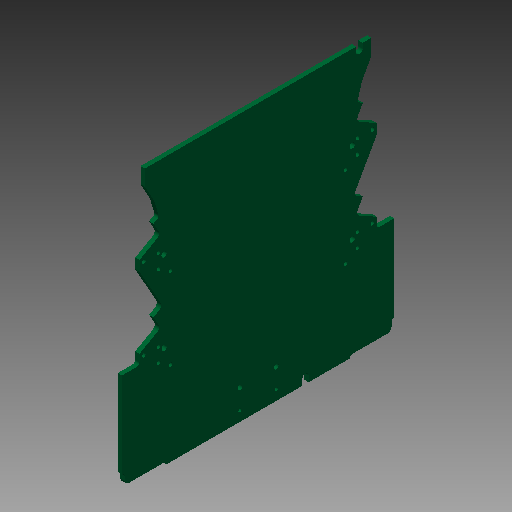
# Autodesk Inventor part: LP CH20M 5.0 2 PCB_5-2
Saved by Autodesk Inventor 2019.3 (Build 233278000, 278)
## iProperties
Category: PARTsolutions
Company: WEIDMUELLER
Created: 2018-11-15
Part Number: LP CH20M 5.0 2 PCB_5-2
Material: Generic
Catalog Web Link: www.cadenas.de
Description: LP CH20M 5.0 2-Elektronikgehäuse
Vendor: WEIDMUELLER
Document SubType Name: Modeling
Designer: psadmin
Manufacturer: WEIDMUELLER
Mass: 13.7336 g
Surface Area: 180.42 cm^2
Volume: 13.7336 cm^3
Density: 1 g/cm^3
Appearance: PSOLRGB-0-127-63
PSOL_IDENT_0: {$CADENAS_DATA\23d-libs\weidmueller\elektronikgehaeuse\einbaugehaeuse\ch20m\zubehoer\lp_ch20m_5_2.pr
PSOL_IDENT_1: j},192 {VTYP=3D},{NB=LP CH20M 5.0 2 PCB_5-2},{LINA=LP CH20M 5.0 2 PCB_5-2},{NN=LP CH20M 5.0 2},{DATE=
PSOL_IDENT_2: 02.11.2012 16:07:47},{GEOMDATE=02.11.2012 16:07:29},{VERSION=},{LINEID=10},{WBVAR=},{WBNUMERIC=}  {N
PSOL_IDENT_3: B=LP CH20M 5.0 2 PCB_5-2},{LINA=LP CH20M 5.0 2 PCB_5-2},{KT=DUMMY},{TYP=PCB_5-2},{BZ=LP CH20M 5.0 2}
PSOL_IDENT_4: ,{FCODE=0.00,0.50,0.25,0.00}
NN: LP CH20M 5.0 2
NT: Elektronikgehäuse
NB: LP CH20M 5.0 2 PCB_5-2
NBSYN: $BZ. $TYP.
LINA: LP CH20M 5.0 2 PCB_5-2
TYP: PCB_5-2
BZ: LP CH20M 5.0 2
FCODE: 0.00,0.50,0.25,0.00
SUPPLIER: WEIDMUELLER
ARTICLENO: LP CH20M 5.0 2 PCB_5-2
BOMINFO: LP CH20M 5.0 2 PCB_5-2
CREATOR: CADENAS GmbH
Title: LP CH20M 5.0 2 PCB_5-2
Author: Cadenas PARTsolutions
Comments: Elektronikgehäuse
Autodesk Inventor part; units mm, degrees
sketch "Sketch_2" plane through (0, 0, 0) normal (1, 0, 0) x (0, 1, 0)
  arc A0 (6, 49.5) -> (7, 50.5) centre (6, 50.5) ccw
  line L0 (6, 49.5) -> (4.5, 49.5)
  arc A1 (4.5, 49.5) -> (3, 48) centre (4.5, 48) ccw
  line L1 (3, 48) -> (3, 35)
  arc A2 (2, 34) -> (3, 35) centre (2, 35) ccw
  line L2 (2, 34) -> (2, -15.6072)
  line L3 (2, -15.6072) -> (2.4, -16.3)
  line L4 (2.4, -16.3) -> (4.2, -16.3)
  arc A3 (4.2, -18.7) -> (4.2, -16.3) centre (4.2, -17.5) ccw
  line L5 (4.2, -18.7) -> (2, -18.7)
  line L6 (2, -18.7) -> (2, -34)
  arc A4 (3, -35) -> (2, -34) centre (2, -35) ccw
  line L7 (3, -35) -> (3, -48)
  arc A5 (3, -48) -> (4.5, -49.5) centre (4.5, -48) ccw
  line L8 (4.5, -49.5) -> (6, -49.5)
  arc A6 (7, -50.5) -> (6, -49.5) centre (6, -50.5) ccw
  line L9 (7, -50.5) -> (38.7662, -50.5)
  line L10 (38.7662, -50.5) -> (38.7662, -45)
  arc A7 (39.7662, -44) -> (38.7662, -45) centre (39.7662, -45) ccw
  line L11 (39.7662, -44) -> (42.5044, -44)
  line L12 (42.5044, -44) -> (46.1424, -37.5038)
  arc A8 (48.1841, -36.928) -> (46.1424, -37.5038) centre (47.4512, -38.2367) ccw
  line L13 (48.1841, -36.928) -> (51.6116, -38.8475)
  line L14 (51.6116, -38.8475) -> (52.8016, -36.7226)
  arc A9 (54.8433, -36.1468) -> (52.8016, -36.7226) centre (54.1103, -37.4555) ccw
  line L15 (54.8433, -36.1468) -> (68.8661, -44)
  line L16 (68.8661, -44) -> (72.6044, -44)
  line L17 (72.6044, -44) -> (76.2424, -37.5038)
  arc A10 (78.2841, -36.928) -> (76.2424, -37.5038) centre (77.5512, -38.2367) ccw
  line L18 (78.2841, -36.928) -> (81.7116, -38.8475)
  line L19 (81.7116, -38.8475) -> (82.4858, -37.4651)
  arc A11 (82.7791, -37.1385) -> (82.4858, -37.4651) centre (83.3583, -37.9537) ccw
  arc A12 (83.6381, -36.9937) -> (82.7791, -37.1385) centre (83.3583, -37.9537) ccw
  line L20 (83.6381, -36.9937) -> (88.8034, -38.4993)
  arc A13 (89.1166, -38.6306) -> (88.8034, -38.4993) centre (88.3836, -39.9393) ccw
  line L21 (89.1166, -38.6306) -> (95.1331, -42)
  line L22 (95.1331, -42) -> (101, -42)
  line L23 (101, -42) -> (101, -38.75)
  line L24 (101, -38.75) -> (99.2, -38.75)
  arc A14 (98.4063, -38.45) -> (99.2, -38.75) centre (99.2, -37.55) ccw
  arc A15 (98.4063, -36.65) -> (98.4063, -38.45) centre (99.2, -37.55) ccw
  arc A16 (99.2, -36.35) -> (98.4063, -36.65) centre (99.2, -37.55) ccw
  line L25 (99.2, -36.35) -> (101, -36.35)
  line L26 (101, -36.35) -> (101, 42)
  line L27 (101, 42) -> (95.1331, 42)
  line L28 (95.1331, 42) -> (89.1166, 38.6306)
  arc A17 (88.8034, 38.4993) -> (89.1166, 38.6306) centre (88.3836, 39.9393) ccw
  line L29 (88.8034, 38.4993) -> (83.6381, 36.9937)
  arc A18 (82.7791, 37.1385) -> (83.6381, 36.9937) centre (83.3583, 37.9537) ccw
  arc A19 (82.4858, 37.4651) -> (82.7791, 37.1385) centre (83.3583, 37.9537) ccw
  line L30 (82.4858, 37.4651) -> (81.7116, 38.8475)
  line L31 (81.7116, 38.8475) -> (78.2841, 36.928)
  arc A20 (76.2424, 37.5038) -> (78.2841, 36.928) centre (77.5512, 38.2367) ccw
  line L32 (76.2424, 37.5038) -> (72.6044, 44)
  line L33 (72.6044, 44) -> (68.8661, 44)
  line L34 (68.8661, 44) -> (54.8433, 36.1468)
  arc A21 (52.8016, 36.7226) -> (54.8433, 36.1468) centre (54.1103, 37.4555) ccw
  line L35 (52.8016, 36.7226) -> (51.6116, 38.8475)
  line L36 (51.6116, 38.8475) -> (48.1841, 36.928)
  arc A22 (46.1424, 37.5038) -> (48.1841, 36.928) centre (47.4512, 38.2367) ccw
  line L37 (46.1424, 37.5038) -> (42.5044, 44)
  line L38 (42.5044, 44) -> (39.7662, 44)
  arc A23 (38.7662, 45) -> (39.7662, 44) centre (39.7662, 45) ccw
  line L39 (38.7662, 45) -> (38.7662, 50.5)
  line L40 (38.7662, 50.5) -> (7, 50.5)
  circle A24 centre (41.2057, -42.3862) radius 0.7
  circle A25 centre (71.3057, -42.3862) radius 0.7
  circle A26 centre (41.1709, -36.9226) radius 0.7
  circle A27 centre (71.2709, -36.9226) radius 0.7
  circle A28 centre (35.9795, -36.8806) radius 0.7
  circle A29 centre (66.0795, -36.8806) radius 0.7
  circle A30 centre (39.7889, -34.8879) radius 1
  circle A31 centre (69.8889, -34.8879) radius 1
  circle A32 centre (33.2312, -32.4762) radius 0.7
  circle A33 centre (63.3312, -32.4762) radius 0.7
  circle A34 centre (5.71, -6.75) radius 0.6
  circle A35 centre (13.01, -6.75) radius 0.9
  circle A36 centre (5.71, 6.75) radius 0.6
  circle A37 centre (13.01, 6.75) radius 0.9
  circle A38 centre (63.3312, 32.4762) radius 0.7
  circle A39 centre (33.2312, 32.4762) radius 0.7
  circle A40 centre (69.8889, 34.8879) radius 1
  circle A41 centre (39.7889, 34.8879) radius 1
  circle A42 centre (66.0795, 36.8806) radius 0.7
  circle A43 centre (35.9795, 36.8806) radius 0.7
  circle A44 centre (71.2709, 36.9226) radius 0.7
  circle A45 centre (41.1709, 36.9226) radius 0.7
  circle A46 centre (71.3057, 42.3862) radius 0.7
  circle A47 centre (41.2057, 42.3862) radius 0.7
  constraints: 82 end point, 48 centre point, 48 point on circle
extrude "Extrusion1" add sketch "Sketch_2" along normal blind 1.6
ref_plane "LPmitBASE_XY" through (0, 0, 0) normal (1, 0, 0) x (0, 0, -1)
ref_plane "LPmitBASE_YZ" through (0, 0, 0) normal (0, 0, -1) x (0, 1, 0)
ref_plane "LPmitBASE_ZX" through (0, 0, 0) normal (0, 1, 0) x (1, 0, 0)
ref_plane "mitSHL01_XY" through (0, 41.2057, -42.3862) normal (1, 0, 0) x (0, 0, -1)
ref_plane "mitSHL01_YZ" through (0, 41.2057, -42.3862) normal (0, 0, -1) x (0, 1, 0)
ref_plane "mitSHL01_ZX" through (0, 41.2057, -42.3862) normal (0, 1, 0) x (1, 0, 0)
ref_plane "mitSHL02_XY" through (0, 71.3057, -42.3862) normal (1, 0, 0) x (0, 0, -1)
ref_plane "mitSHL02_YZ" through (0, 71.3057, -42.3862) normal (0, 0, -1) x (0, 1, 0)
ref_plane "mitSHL02_ZX" through (0, 71.3057, -42.3862) normal (0, 1, 0) x (1, 0, 0)
ref_plane "mitSHL03_XY" through (0, 41.2057, 42.3862) normal (1, 0, 0) x (0, 0, -1)
ref_plane "mitSHL03_YZ" through (0, 41.2057, 42.3862) normal (0, 0, -1) x (0, 1, 0)
ref_plane "mitSHL03_ZX" through (0, 41.2057, 42.3862) normal (0, 1, 0) x (1, 0, 0)
ref_plane "mitSHL04_XY" through (0, 71.3057, 42.3862) normal (1, 0, 0) x (0, 0, -1)
ref_plane "mitSHL04_YZ" through (0, 71.3057, 42.3862) normal (0, 0, -1) x (0, 1, 0)
ref_plane "mitSHL04_ZX" through (0, 71.3057, 42.3862) normal (0, 1, 0) x (1, 0, 0)
body "Solid1"
